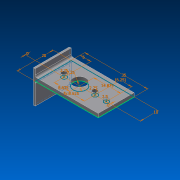
# Autodesk Inventor part: tac switch test
Saved by Autodesk Inventor 2015 (Build 190159000, 159)
## iProperties
Created: 2017-03-16
Part Number: tac switch test
Material: Generic
Document SubType Name: Modeling
Designer: ZigZagJoe
Density: 1 g/cm^3
Appearance: Default
Author: ZigZagJoe
Autodesk Inventor part; units mm, degrees
ref_plane "YZ Plane" through (0, 0, 0) normal (1, 0, 0) x (0, 1, 0)
ref_plane "XZ Plane" through (0, 0, 0) normal (0, 1, 0) x (-1, 0, 0)
ref_plane "XY Plane" through (0, 0, 0) normal (0, 0, 1) x (1, 0, 0)
sketch "Sketch1" plane through (0, 0, 0) normal (0, 0, 1) x (1, 0, 0)
  line L0 (-12.9399, 8.8675) -> (22.0601, 8.8675)
  line L1 (22.0601, 8.8675) -> (22.0601, -11.1325)
  line L2 (22.0601, -11.1325) -> (-12.9399, -11.1325)
  line L3 (-12.9399, -11.1325) -> (-12.9399, 8.8675)
  circle A0 centre (-6.9399, -1.1325) radius 1.375
  circle A1 centre (10.3101, -1.1325) radius 1.375
  circle A2 centre (1.6851, -1.1325) radius 3.625
  circle A3 centre (16.5601, -1.1325) radius 1.25
  point P0 (0, 0)
  dimension "d0" = 20
  dimension "d1" = 35
  dimension "d2" = 7.25
  dimension "d3" = 2.75
  dimension "d4" = 2.75
  dimension "d5" = 8.625
  dimension "d6" = 0
  dimension "d7" = 8.625
  dimension "d8" = 0
  dimension "d9" = 6
  dimension "d10" = 10
  dimension "d20" = 2.5
  dimension "d21" = 14.875
  dimension "d24" = 6.25
  constraints: 8 end point, 4 centre point, 2 parallel, 1 horizontal, 1 perpendicular
  measures "d0" distance of L2.end L0.start
  measures "d1" distance of L0.start L0.end
  measures "d2" diameter of A2
  measures "d3" diameter of A0
  measures "d4" diameter of A1
  measures "d5" distance of A2.centre A0.centre
  measures "d6" vertical distance of A0.centre A2.centre
  measures "d7" distance of A2.centre A1.centre
  measures "d8" vertical distance of A2.centre A1.centre
  measures "d9" distance from line of L3 A0.centre
  measures "d10" distance from line of L0 A2.centre
  measures "d20" diameter of A3
  measures "d21" distance of A3.centre A2.centre
  measures "d24" distance of A1.centre A3.centre
extrude "Extrusion1" add sketch "Sketch1" along normal blind 2 contours L0 L1 L2 L3 | A3
sketch "Sketch2" plane through (-12.9399, -11.1325, 0) normal (-1, 0, 0) x (0, 0, 1)
  line L0 (-12, 20) -> (6, 20)
  line L1 (6, 20) -> (6, 0)
  line L2 (6, 0) -> (-12, 0)
  line L3 (-12, 0) -> (-12, 20)
  line L4 (0, 0) -> (0, 20) projected
  line L5 (2, 20) -> (2, 0) projected
  point P0 (0, 11.1325)
  dimension "d13" = 12
  dimension "d14" = 4
  dimension "d15" = 0
  dimension "d16" = 0
  constraints: 8 end point, 2 parallel, 1 horizontal, 1 perpendicular
  measures "d13" distance from line of L0.start L4
  measures "d14" distance between parallel lines of L1 L5
  measures "d15" vertical distance of L0.end L5.start
  measures "d16" vertical distance of L1.end L5.end
extrude "Extrusion2" add sketch "Sketch2" along normal blind 1
fillet "Fillet1" radius 1 2 edges at (-12.9399, -1.1325, 2) (-12.9399, -1.1325, 0)
extrude "Extrusion3" cut sketch "Sketch1" along normal blind 1 contours A3
equation "\"d7\" = d5"
body "Solid1"
